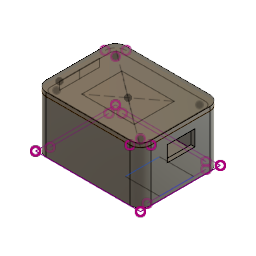
case (Autodesk Fusion 360 design; units mm, degrees)
Autodesk Fusion 360 part; units mm, degrees
sketch "Base" plane through (0, 0, 0) normal (0, 1, 0) x (1, 0, 0) in component "Top"
  line L0 (0, 0) -> (40, 0)
  line L1 (40, 0) -> (40, 30.5)
  line L2 (40, 30.5) -> (0, 30.5)
  line L3 (0, 30.5) -> (0, 0)
  dimension "d6" = 40
  dimension "d7" = 30.5
  constraint horizontal L0
  constraint vertical L1
  constraint horizontal L2
  constraint vertical L3
  constraint coincident L0.start L3.end
  measures "d6" distance of L0.start L0.end
  measures "d7" distance of L0.start L2.end
extrude "Extrude1" add sketch "Base" along normal blind 20 makes body 1 in component "Top"
fillet "Fillet1" radius 4 4 edges at (40, 10, 0) (0, 10, 0) (40, 10, -30.5) (0, 10, -30.5) on bodies 1 in component "Top"
shell "Shell1" thickness 1.5 removed faces 1 at (25.3333, 20, -10.1667) on bodies 1 in component "Top"
sketch "Knob" plane through (1.5, 0, 0) normal (1, 0, 0) x (0, 0, -1) in component "Top"
  line L0 (26.5, 1.5) -> (26.5, 20)
  line L1 (26.5, 20) -> (4, 20)
  line L2 (4, 20) -> (4, 1.5)
  line L3 (4, 1.5) -> (26.5, 1.5)
  line L4 (7.625, 20) -> (22.875, 20)
  line L5 (22.875, 20) -> (22.875, 17)
  line L6 (22.875, 17) -> (7.625, 17)
  line L7 (7.625, 17) -> (7.625, 20)
  line L8 (15.25, 20) -> (15.25, 17) construction
  dimension "d12" = 15.25
  dimension "d13" = 3
  constraint horizontal L4
  constraint vertical L5
  constraint horizontal L6
  constraint vertical L7
  constraint coincident L1 L4.start
  constraint midpoint L1 L8.start
  constraint midpoint L6 L8.end
  constraint vertical L8
  measures "d12" distance of L5.end L6.end
  measures "d13" distance of L4.end L5.end
extrude "Extrude2" add sketch "Knob" along normal blind 6 draft -45 contours L1 L4 L5 L6 L7 bodies 1 in component "Top"
ref_plane "WorkPlane2" through (20, 10, -15.25) normal (-1, 0, 0) x (0, 0, 1) in component "Top"
mirror "Mirror1" about plane through (20, 10, -15.25) normal (-1, 0, 0) of "Extrude2" in component "Top"
sketch "Top" plane through (0, 20, 0) normal (0, 1, 0) x (-1, 0, 0) in component "Base"
  line L0 (-40, -4) -> (-40, -26.5)
  arc A0 (-40, -26.5) -> (-36, -30.5) centre (-36, -26.5) ccw
  line L1 (-36, -30.5) -> (-4, -30.5)
  arc A1 (-4, -30.5) -> (0, -26.5) centre (-4, -26.5) ccw
  line L2 (0, -26.5) -> (0, -4)
  arc A2 (0, -4) -> (-4, 0) centre (-4, -4) ccw
  line L3 (-4, 0) -> (-36, 0)
  arc A3 (-36, 0) -> (-40, -4) centre (-36, -4) ccw
  line L4 (-38.5, -7.625) -> (-38.5, -4)
  arc A4 (-36, -1.5) -> (-38.5, -4) centre (-36, -4) ccw
  line L5 (-36, -1.5) -> (-4, -1.5)
  arc A5 (-1.5, -4) -> (-4, -1.5) centre (-4, -4) ccw
  line L6 (-1.5, -4) -> (-1.5, -7.625)
  line L7 (-1.5, -7.625) -> (-1.5, -22.875)
  line L8 (-1.5, -22.875) -> (-1.5, -26.5)
  arc A6 (-4, -29) -> (-1.5, -26.5) centre (-4, -26.5) ccw
  line L9 (-4, -29) -> (-36, -29)
  arc A7 (-38.5, -26.5) -> (-36, -29) centre (-36, -26.5) ccw
  line L10 (-38.5, -26.5) -> (-38.5, -22.875)
  line L11 (-38.5, -22.875) -> (-38.5, -7.625)
extrude "Extrude1'" add sketch "Top" along normal blind 1.5 separate body contours L0 A0 L1 A1 L2 A2 L3 A3 | L4 A4 L5 A5 L6 L7 L8 A6 L9 A7 L10 L11 makes body 2 in component "Base"
sketch "Lip" plane through (0, 20, 0) normal (0, -1, 0) x (1, 0, 0) in component "Base"
  arc A0 (40, -4) -> (36, 0) centre (36, -4) ccw
  line L0 (36, 0) -> (4, 0)
  arc A1 (4, 0) -> (0, -4) centre (4, -4) ccw
  line L1 (0, -4) -> (0, -26.5)
  arc A2 (0, -26.5) -> (4, -30.5) centre (4, -26.5) ccw
  line L2 (4, -30.5) -> (36, -30.5)
  arc A3 (36, -30.5) -> (40, -26.5) centre (36, -26.5) ccw
  line L3 (40, -26.5) -> (40, -4)
  line L4 (38.3, -26.5) -> (38.3, -4)
  arc A4 (38.3, -4) -> (36, -1.7) centre (36, -4) ccw
  line L5 (36, -1.7) -> (4, -1.7)
  arc A5 (4, -1.7) -> (1.7, -4) centre (4, -4) ccw
  line L6 (1.7, -4) -> (1.7, -26.5)
  arc A6 (1.7, -26.5) -> (4, -28.8) centre (4, -26.5) ccw
  line L7 (4, -28.8) -> (36, -28.8)
  arc A7 (36, -28.8) -> (38.3, -26.5) centre (36, -26.5) ccw
  dimension "d19" = 1.7
extrude "Extrude2'" add sketch "Lip" along normal blind 3 contours L4 A4 L5 A5 L6 A6 L7 A7 bodies 2 in component "Base"
extrude "Extrude3" cut sketch "Knob" along normal blind 3 draft -45 from surface at 0.2 contours L1 L4 L5 L6 L7 bodies 2 in component "Base"
mirror "Mirror1'" about plane through (20, 10, -15.25) normal (-1, 0, 0) of "Extrude3" in component "Base"
shell "Shell1'" thickness 1.5 removed faces 1 at (13.9, 17, -17.7917) on bodies 2 in component "Base"
chamfer "Chamfer1" distance 0.6 angle 45 2 edges at (1.7, 17, -15.25) (38.3, 17, -15.25) on bodies 2 in component "Base"
sketch "PCB Mount" plane through (0, 20, 0) normal (0, -1, 0) x (1, 0, 0) in component "Base"
  arc A0 (40, -4) -> (36, 0) centre (36, -4) ccw construction
  arc A1 (0, -26.5) -> (4, -30.5) centre (4, -26.5) ccw construction
  line L0 (38.8284, -1.1716) -> (1.1716, -29.3284) construction
  line L1 (30, -22.875) -> (10, -22.875)
  line L2 (10, -22.875) -> (10, -7.625)
  line L3 (10, -7.625) -> (30, -7.625)
  line L4 (30, -7.625) -> (30, -22.875)
  line L5 (30, -22.875) -> (10, -7.625) construction
  line L6 (10, -22.875) -> (30, -7.625) construction
  point P0 (20, -15.25)
  dimension "d33" = 20
  dimension "d34" = 15.25
  constraint midpoint A0 L0.start
  constraint midpoint A1 L0.end
  constraint perpendicular L1 L2
  constraint parallel L1 L3
  constraint parallel L2 L4
  constraint horizontal L1
  constraint coincident L5 P0
  constraint coincident L6 P0
  constraint midpoint L0 P0
  measures "d33" distance of L2.end L3.end
  measures "d34" distance of L1.end L2.end
sketch "Right Holes" plane through (40, 0, 0) normal (1, 0, 0) x (0, 0, -1) in component "Top"
  line L0 (26.5, 20) -> (4, 20)
  line L1 (4, 20) -> (4, 0)
  line L2 (4, 0) -> (26.5, 0)
  line L3 (26.5, 0) -> (26.5, 20)
  line L4 (0, 20) -> (0, 0)
  line L5 (0, 0) -> (30.5, 0)
  line L6 (7.625, 20) -> (22.875, 20)
  line L7 (10.25, 11) -> (20.75, 11)
  line L8 (20.75, 11) -> (20.75, 17)
  line L9 (20.75, 17) -> (10.25, 17)
  line L10 (10.25, 17) -> (10.25, 11)
  dimension "d75" = 10.5
  dimension "d76" = 6
  dimension "d81" = 3
  dimension "d82" = 10.25
  constraint horizontal L7
  constraint vertical L8
  constraint horizontal L9
  constraint vertical L10
  measures "d75" distance of L7.start L7.end
  measures "d76" distance of L7.start L9.end
  measures "d81" distance of L0 L9
  measures "d82" distance of L4 L10
sketch "Top Holes" plane through (0, 0, 0) normal (0, 1, 0) x (1, 0, 0) in component "Top"
  line L0 (0, 30.5) -> (0, 0)
  line L1 (40, 30.5) -> (0, 30.5)
  line L2 (0, 0) -> (40, 0)
  line L3 (40, 0) -> (40, 30.5)
  line L4 (25.5, 21.75) -> (38.5, 21.75)
  line L5 (38.5, 21.75) -> (38.5, 8.75)
  line L6 (38.5, 8.75) -> (25.5, 8.75)
  line L7 (25.5, 8.75) -> (25.5, 21.75)
  line L8 (36, 29) -> (4, 29)
  line L9 (1.5, 4) -> (1.5, 26.5)
  line L10 (38.5, 4) -> (38.5, 26.5)
  dimension "d55" = 13
  dimension "d58" = 13
  dimension "d80" = 8.75
  constraint horizontal L4
  constraint vertical L5
  constraint horizontal L6
  constraint vertical L7
  measures "d55" distance of L4.end L5.end
  measures "d58" distance of L5 L7
  measures "d80" distance of L1 L4
extrude "Extrude5" cut sketch "Top Holes" along normal blind 3 contours L4 L5 L6 L7 L10 bodies 1 in component "Top"
extrude "Extrude10" cut sketch "Right Holes" against normal up to surface (1.5 mm away) contours L7 L8 L9 L10 bodies 1 in component "Top"
component "Enclosure" placed x (1, 0, 0) y (0, 1, 0) z (0, 0, 1) at (0, 0, 0)
component "Top" placed x (1, 0, 0) y (0, 1, 0) z (0, 0, 1) at (0, 0, 0) in component "Enclosure"
component "Base" placed x (1, 0, 0) y (0, 1, 0) z (0, 0, 1) at (0, 0, 0) in component "Enclosure"
equation "Width = 30.5 mm"
equation "length = 40 mm"
equation "heigth = 20 mm"
equation "shell = 1.5 mm"
equation "gap = 0.2 mm"
equation "d6 = length"
equation "d7 = Width"
equation "d8 = heigth"
equation "d11 = shell"
equation "d12 = Width / 2"
equation "d13 = shell * 2"
equation "d17 = shell"
equation "d19 = shell + gap"
equation "d20 = shell * 2"
equation "d23 = shell * 2"
equation "d26 = shell"
equation "d33 = length / 2"
equation "d34 = Width / 2"
equation "d80 = ( Width / 2 ) - 6.5 mm"
equation "d82 = ( Width / 2 ) - 5 mm"
